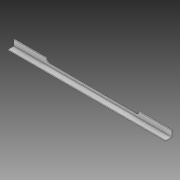
# Autodesk Inventor part: FE-120-001 Floor L Section
Saved by Autodesk Inventor 2021 (Build 250183000, 183)
## iProperties
Created: 2021-01-11
Part Number: FE-120-001 Floor L Section
Material: Aluminum 6061
Document SubType Name: Modeling
Density: 2.7 g/cm^3
Appearance: Aluminum - Dark
Autodesk Inventor part; units mm, degrees
ref_plane "YZ Plane" through (0, 0, 0) normal (1, 0, 0) x (0, 1, 0)
ref_plane "XZ Plane" through (0, 0, 0) normal (0, 1, 0) x (-1, 0, 0)
ref_plane "XY Plane" through (0, 0, 0) normal (0, 0, 1) x (1, 0, 0)
sketch "Sketch1" plane through (0, 0, 0) normal (1, 0, 0) x (0, 1, 0)
  line L0 (0, 0) -> (76.2, 0)
  line L1 (0, 0) -> (0, 76.2)
  arc A0 (6.35, 71.12) -> (1.27, 76.2) centre (1.27, 71.12) ccw
  arc A1 (76.2, 1.27) -> (71.12, 6.35) centre (71.12, 1.27) ccw
  line L2 (76.2, 0) -> (76.2, 1.27)
  line L3 (1.27, 76.2) -> (0, 76.2)
  arc A2 (6.35, 11.43) -> (11.43, 6.35) centre (11.43, 11.43) ccw
  line L4 (6.35, 71.12) -> (6.35, 11.43)
  line L5 (11.43, 6.35) -> (71.12, 6.35)
  dimension "d0" = 76.2
  dimension "d1" = 76.2
  dimension "d2" = 10.16
  dimension "d3" = 10.16
  dimension "d4" = 10.16
  dimension "d5" = 6.35
  constraints: 12 end point, 6 perpendicular, 6 point on circle, 5 tangent, 3 centre point, 1 horizontal, 1 vertical
  measures "d0" distance of L0.start L0.end
  measures "d1" distance of L0.start L1.end
  measures "d2" diameter of A0
  measures "d3" diameter of A1
  measures "d4" diameter of A2
  measures "d5" distance between parallel lines of L1 L4
extrude "Extrusion1" add sketch "Sketch1" along normal mid plane 1828.8
sketch "Sketch2" plane through (-914.4, 11.43, 6.35) normal (0, 0, 1) x (1, 0, 0)
  line L0 (381, 26.67) -> (1447.8, 26.67)
  line L1 (1447.8, 26.67) -> (1447.8, 64.77)
  line L2 (1447.8, 64.77) -> (381, 64.77)
  line L3 (381, 64.77) -> (381, 26.67)
  line L4 (381, 26.67) -> (1447.8, 64.77) construction
  line L5 (1447.8, 26.67) -> (381, 64.77) construction
  line L6 (0, 64.77) -> (1828.8, 64.77) projected
  line L7 (1828.8, -10.16) -> (0, -10.16) projected
  point P0 (914.4, -11.43)
  point P1 (914.4, 45.72)
  point P2 (914.4, 45.72)
  point P3 (914.4, -10.16)
  dimension "d8" = 1066.8
  dimension "d9" = 38.1
  constraints: 12 end point, 4 midpoint, 2 parallel, 1 collinear, 1 horizontal, 1 perpendicular, 1 vertical alignment
  measures "d8" distance of L2.end L1.end
  measures "d9" distance of L1.end L0.end
extrude "Extrusion2" cut sketch "Sketch2" against normal through all
fillet "Fillet1" radius 25.4 2 edges at (-533.4, 38.1, 3.175) (533.4, 38.1, 3.175)
body "Solid1"
